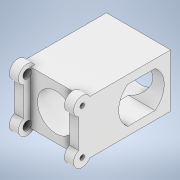
# Autodesk Inventor part: MotorMount
Saved by Autodesk Inventor 2022 (Build 260153000, 153)
## iProperties
Created: 2022-02-05
Part Number: MotorMount
Material: Generic
Document SubType Name: Modeling
Designer: ultra
Density: 1 g/cm^3
Appearance: Smooth - White
Author: ultra
Autodesk Inventor part; units mm, degrees
ref_plane "YZ Plane" through (0, 0, 0) normal (1, 0, 0) x (0, 1, 0)
ref_plane "XZ Plane" through (0, 0, 0) normal (0, 1, 0) x (-1, 0, 0)
ref_plane "XY Plane" through (0, 0, 0) normal (0, 0, 1) x (1, 0, 0)
sketch "Sketch1" plane through (0, 0, 0) normal (1, 0, 0) x (0, 1, 0)
  arc A0 (-5.7904, 15.7173) -> (3.1801, 16.4454) centre (0, 0) ccw
  line L0 (3.6239, 10.9763) -> (3.1801, 16.4454)
  line L1 (-5.3466, 10.2483) -> (3.6239, 10.9763)
  line L2 (-5.7904, 15.7173) -> (-5.3466, 10.2483)
  circle A1 centre (8.6526, -9.0212) radius 1.5
  circle A2 centre (-9.0212, -8.6526) radius 1.5
  circle A3 centre (-8.6526, 9.0212) radius 1.5
  circle A4 centre (9.0212, 8.6526) radius 1.5
  circle A5 centre (0, 0) radius 6.8
  circle A6 centre (8.6526, -9.0212) radius 1.5875
  circle A7 centre (-9.0212, -8.6526) radius 1.5875
  circle A8 centre (-8.6526, 9.0212) radius 1.5875
  circle A9 centre (9.0212, 8.6526) radius 1.5875
  circle A10 centre (0, 0) radius 16.75
  point P0 (-5.7904, 15.7173)
  point P1 (3.1801, 16.4454)
  dimension "d2" = 3.175
  dimension "d3" = 3.175
  dimension "d4" = 3.175
  dimension "d5" = 3.175
  constraints: 11 centre point, 6 end point, 5 coincident, 2 point on circle, 1 concentric
  measures "d2" diameter of A6
  measures "d3" diameter of A7
  measures "d4" diameter of A8
  measures "d5" diameter of A9
extrude "Extrusion3" add sketch "Sketch1" along normal blind 6.35 contours L2 L1 L0 A0 | A10 L0 L1 L2
sketch "Sketch4" plane through (6.35, 0, 0) normal (1, 0, 0) x (0, 0, -1)
  circle A0 centre (0, 0) radius 16.75 projected
  circle A1 centre (-25.4, 0) radius 6.35
  circle A2 centre (0, 0) radius 6.35
  circle A3 centre (-38.7858, -15.6249) radius 2.925
  circle A4 centre (-38.7858, 15.6249) radius 2.925
  line L0 (-41.275, 10.1656) -> (-41.275, -10.1656)
  arc A5 (-41.275, -10.1656) -> (-33.5216, -18.5039) centre (-38.7858, -15.6249) ccw
  line L1 (-33.5216, -18.5039) -> (20.3643, -18.5039)
  line L2 (-33.5216, 18.5039) -> (9.525, 18.5039)
  arc A6 (-33.5216, 18.5039) -> (-41.275, 10.1656) centre (-38.7858, 15.6249) ccw
  line L3 (20.3643, -18.5039) -> (20.3643, 18.5039)
  line L4 (20.3643, 18.5039) -> (8.806, 18.5039)
  point P0 (-41.275, 18.5039)
  constraints: 10 end point, 6 centre point, 4 point on circle, 1 point on line, 1 vertical
extrude "Extrusion5" add sketch "Sketch4" along normal blind 41.5544 contours A6 L2 L4 L3 L1 A5 L0
sketch "Sketch5" plane through (6.35, -18.5039, -20.3643) normal (0, 0, -1) x (-1, 0, 0)
  circle A0 centre (-20.7772, 18.5039) radius 12.8778
  point P0 (6.35, 18.5039)
  dimension "d22" = 25.7556
  constraints: 1 centre point
  measures "d22" diameter of A0
extrude "Extrusion6" cut sketch "Sketch5" against normal up to surface (61.6393 mm away)
sketch "Sketch6" plane through (6.35, 0, 0) normal (-1, 0, 0) x (0, 0, 1)
  circle A0 centre (25.4, 0) radius 6.35 projected
  circle A1 centre (38.7858, -15.6249) radius 2.925 projected
  circle A2 centre (38.7858, 15.6249) radius 2.925 projected
  line L0 (55.9002, 27.2812) -> (18.3497, 27.2812)
  line L1 (18.3497, 27.2812) -> (18.3497, -27.035)
  line L2 (18.3497, -27.035) -> (55.9002, -27.035)
  line L3 (55.9002, -27.035) -> (55.9002, 27.2812)
  constraints: 8 end point, 2 parallel, 1 horizontal, 1 perpendicular
extrude "Extrusion7" cut sketch "Sketch6" against normal blind 76.2
sketch "Sketch7" plane through (6.35, -18.5039, 18.3497) normal (0, 0, 1) x (1, 0, 0)
  line L0 (41.5544, 0) -> (0, 0) projected
  line L1 (41.5544, 37.0078) -> (41.5544, 0) projected
  line L2 (0, 37.0078) -> (41.5544, 37.0078) projected
  line L3 (0, 0) -> (0, 37.0078) projected
  circle A0 centre (20.7772, 18.5039) radius 12.8778 projected
  point P0 (-6.35, 18.5039)
extrude "Extrusion8" add sketch "Sketch7" along normal blind 25.4
sketch "Sketch8" plane through (6.35, 0, 0) normal (-1, 0, 0) x (0, 0, 1)
  line L0 (43.7497, -18.5039) -> (-17.8897, -18.5039)
  line L1 (43.7497, 18.5039) -> (43.7497, -18.5039)
  line L2 (-7.0503, 18.5039) -> (43.7497, 18.5039)
  line L3 (-25.5542, 0.0039) -> (43.7497, 0.0039)
  line L4 (43.7497, 12.8817) -> (43.7497, -12.8739)
  circle A0 centre (41.2605, -15.6249) radius 1.5875
  circle A1 centre (41.2605, 15.6249) radius 1.5875
  dimension "d29" = 3.175
  dimension "d30" = 3.175
  dimension "d31" = 2.7432
  dimension "d32" = 2.4892
  dimension "d33" = 2.879
  dimension "d34" = 2.879
  constraints: 10 end point, 2 centre point, 1 midpoint
  measures "d29" diameter of A0
  measures "d30" diameter of A1
  measures "d31" vertical distance of L4.start A1.centre
  measures "d32" distance from line of L1 A0.centre
  measures "d33" distance from line of L0 A0.centre
  measures "d34" distance from line of L2 A1.centre
extrude "Extrusion9" cut sketch "Sketch8" against normal blind 50.8
sketch "Sketch9" plane through (0, 0, 0) normal (-1, 0, 0) x (0, 0, 1)
  circle A0 centre (0, 0) radius 16.75 projected
  circle A1 centre (8.6526, 9.0212) radius 1.5875 projected
  circle A2 centre (9.0212, -8.6526) radius 1.5875 projected
  circle A3 centre (-8.6526, -9.0212) radius 1.5875 projected
  circle A4 centre (-9.0212, 8.6526) radius 1.5875 projected
  circle A5 centre (0, 0) radius 6.8 projected
sketch "Sketch10" plane through (6.35, 0, 0) normal (-1, 0, 0) x (0, 0, 1)
  circle A0 centre (41.2605, 15.6249) radius 1.5875 projected
  circle A1 centre (41.2605, -15.6249) radius 1.5875 projected
  circle A2 centre (0, 0) radius 16.75 projected
  line L0 (-20.3643, 18.5039) -> (43.7497, 18.5039) projected
  line L1 (-20.3643, -18.5039) -> (-20.3643, 18.5039) projected
  line L2 (43.7497, -18.5039) -> (-20.3643, -18.5039) projected
  line L3 (43.7497, 18.5039) -> (43.7497, -18.5039) projected
extrude "Extrusion10" add sketch "Sketch10" along normal blind 3.175
extrude "Extrusion11" cut sketch "Sketch9" against normal blind 3.175
sketch "Sketch11" plane through (6.35, 0, 0) normal (1, 0, 0) x (0, 0, -1)
  circle A0 centre (0, 0) radius 16.75 projected
  circle A1 centre (-8.6526, 9.0212) radius 1.5875 projected
  circle A2 centre (-9.0212, -8.6526) radius 1.5875 projected
  circle A3 centre (8.6526, -9.0212) radius 1.5875 projected
  circle A4 centre (9.0212, 8.6526) radius 1.5875 projected
  circle A5 centre (0, 0) radius 6.8 projected
extrude "Extrusion12" add sketch "Sketch11" along normal blind 3.175
sketch "Sketch12" plane through (3.175, 0, 0) normal (-1, 0, 0) x (0, 0, 1)
  circle A0 centre (41.2605, -15.6249) radius 1.5875 projected
  circle A1 centre (41.2605, 15.6249) radius 1.5875 projected
  circle A2 centre (41.2605, 15.6249) radius 6
  circle A3 centre (41.2605, -15.6249) radius 6
  dimension "d43" = 12
  dimension "d44" = 12
  constraints: 2 centre point, 2 coincident
  measures "d43" diameter of A2
  measures "d44" diameter of A3
sketch "Sketch13" plane through (47.9044, 0, 0) normal (1, 0, 0) x (0, 0, -1)
  circle A0 centre (-41.2605, 15.6249) radius 1.5875 projected
  circle A1 centre (-41.2605, -15.6249) radius 1.5875 projected
  circle A2 centre (-41.2605, -15.6249) radius 6
  circle A3 centre (-41.2605, 15.6249) radius 6
  constraints: 2 centre point, 2 coincident
sketch "Sketch14" plane through (6.35, -18.5039, 43.7497) normal (0, 0, 1) x (1, 0, 0)
  line L0 (36.7792, 28.6695) -> (36.7792, 37.0078) projected
  line L1 (41.5544, 37.0078) -> (-3.175, 37.0078) projected
  line L2 (1.6002, 37.0078) -> (1.6002, 28.6695) projected
  line L3 (1.6002, 28.6695) -> (-3.175, 28.6695) projected
  line L4 (-3.175, 0) -> (-3.175, 37.0078) projected
  line L5 (-3.175, 8.3383) -> (1.6002, 8.3383) projected
  line L6 (1.6002, 8.3383) -> (1.6002, 0) projected
  line L7 (41.5544, 0) -> (-3.175, 0) projected
  line L8 (36.7792, 0) -> (36.7792, 8.3383) projected
  line L9 (36.7792, 8.3383) -> (41.5544, 8.3383) projected
  line L10 (41.5544, 0) -> (41.5544, 37.0078) projected
  line L11 (41.5544, 28.6695) -> (36.7792, 28.6695) projected
  circle A0 centre (20.7772, 18.5039) radius 12.8778 projected
  point P0 (-6.35, 18.5039)
extrude "Extrusion15" cut sketch "Sketch14" against normal blind 5.0038 contours L11 L10 L9 L8 L7 L6 L5 L4 L3 L2 L1 L0
extrude "Extrusion16" add sketch "Sketch13" against normal blind 4.7752
extrude "Extrusion17" add sketch "Sketch12" against normal blind 4.7752
sketch "Sketch15" plane through (3.175, 0, 0) normal (-1, 0, 0) x (0, 0, 1)
  circle A0 centre (41.2605, -15.6249) radius 1.5875 projected
  circle A1 centre (41.2605, 15.6249) radius 1.5875 projected
  arc A2 (38.7713, 10.1656) -> (35.9963, 18.5039) centre (41.2605, 15.6249) ccw projected
  arc A3 (35.9963, -18.5039) -> (38.7713, -10.1656) centre (41.2605, -15.6249) ccw projected
  circle A4 centre (41.2605, -15.6249) radius 2.925
  circle A5 centre (41.2605, 15.6249) radius 2.925
  dimension "d55" = 5.85
  dimension "d56" = 5.85
  constraints: 2 centre point, 2 coincident
  measures "d55" diameter of A4
  measures "d56" diameter of A5
extrude "Extrusion18" cut sketch "Sketch15" against normal blind 6.6675
sketch "Sketch16" plane through (3.175, 0, 0) normal (-1, 0, 0) x (0, 0, 1)
  line L0 (38.7713, -10.1656) -> (38.7459, -10.1656) projected
  line L1 (38.7459, -10.1656) -> (38.7459, 10.1656) projected
  line L2 (38.7459, 10.1656) -> (38.7713, 10.1656) projected
  arc A0 (38.7713, 10.1656) -> (35.9963, 18.5039) centre (41.2605, 15.6249) ccw projected
  arc A1 (35.9963, -18.5039) -> (38.7713, -10.1656) centre (41.2605, -15.6249) ccw projected
  circle A2 centre (41.2605, 15.6249) radius 1.5875
  circle A3 centre (41.2605, -15.6249) radius 1.5875
  line L3 (-20.3643, 18.5039) -> (43.7497, 18.5039)
  line L4 (43.7497, -18.5039) -> (-20.3643, -18.5039)
  line L5 (43.7497, 18.5039) -> (43.7497, -18.5039)
  line L6 (38.7459, -18.5039) -> (35.9963, -18.5039) projected
  line L7 (38.3355, -18.5039) -> (38.3355, 18.5039)
  point P0 (43.7497, -10.1656)
  point P1 (43.7497, 10.1656)
  constraints: 8 end point, 2 centre point, 2 point on line, 1 perpendicular
extrude "Extrusion19" add sketch "Sketch16" against normal blind 4.7752 contours L0 L1 L2 A0 L5 A1
sketch "Sketch17" plane through (47.9044, 0, 0) normal (1, 0, 0) x (0, 0, -1)
  line L0 (-38.7713, 10.1656) -> (-38.7459, 10.1656) projected
  line L1 (-38.7459, 10.1656) -> (-38.7459, -10.1656) projected
  line L2 (-38.7459, -10.1656) -> (-38.7713, -10.1656) projected
  arc A0 (-38.7713, -10.1656) -> (-35.9963, -18.5039) centre (-41.2605, -15.6249) ccw projected
  arc A1 (-35.9963, 18.5039) -> (-38.7713, 10.1656) centre (-41.2605, 15.6249) ccw projected
  circle A2 centre (-41.2605, -15.6249) radius 1.5875
  circle A3 centre (-41.2605, 15.6249) radius 1.5875
  line L3 (20.3643, -18.5039) -> (-43.7497, -18.5039)
  line L4 (-43.7497, 18.5039) -> (20.3643, 18.5039)
  line L5 (-43.7497, -18.5039) -> (-43.7497, 18.5039)
  point P0 (-43.7497, 10.1656)
  point P1 (-43.7497, -10.1656)
  constraints: 6 end point, 2 centre point
extrude "Extrusion20" add sketch "Sketch17" against normal blind 4.7752 contours L0 L1 L2 A0 L5 A1
sketch "Sketch18" plane through (7.9502, 18.5039, 38.7459) normal (1, 0, 0) x (0, 0, -1)
  arc A0 (0, -32.6347) -> (0, -35.6229) centre (-2.5146, -34.1288) ccw projected
  arc A1 (0, -1.3849) -> (0, -4.3731) centre (-2.5146, -2.879) ccw projected
  line L0 (0, -1.3849) -> (0, 0) projected
  line L1 (2.7496, 0) -> (0, 0) projected
  arc A2 (2.7496, 0) -> (-5.0038, -8.3383) centre (-2.5146, -2.879) ccw projected
  line L2 (-5.0038, -8.3383) -> (-5.0038, -28.6695) projected
  arc A3 (-5.0038, -28.6695) -> (2.7496, -37.0078) centre (-2.5146, -34.1288) ccw projected
  line L3 (0, -37.0078) -> (2.7496, -37.0078) projected
  line L4 (0, -37.0078) -> (0, -4.3731) projected
  point P0 (38.7459, -18.5039)
  point P1 (0, -32.6347)
sketch "Sketch19" plane through (43.1292, -18.5039, 38.7459) normal (-1, 0, 0) x (0, 0, 1)
  circle A0 centre (2.5146, 2.879) radius 1.5875 projected
  circle A1 centre (2.5146, 34.1288) radius 1.5875 projected
  line L0 (0, 37.0078) -> (0, 0) projected
  line L1 (-2.7496, 0) -> (0, 0) projected
  arc A2 (-2.7496, 0) -> (5.0038, 8.3383) centre (2.5146, 2.879) ccw projected
  line L2 (5.0038, 8.3383) -> (5.0038, 28.6695) projected
  arc A3 (5.0038, 28.6695) -> (-2.7496, 37.0078) centre (2.5146, 34.1288) ccw projected
  line L3 (0, 37.0078) -> (-2.7496, 37.0078) projected
  point P0 (-38.7459, 18.5039)
extrude "Extrusion22" add sketch "Sketch19" along normal blind 1.5875
extrude "Extrusion23" add sketch "Sketch18" along normal blind 1.5875 contours A0 L4 L3 A3 L2 A2 L1 L0 A1
sketch "Sketch20" plane through (9.525, 0, 0) normal (1, 0, 0) x (0, 0, -1)
  circle A0 centre (0, 0) radius 16.75 projected
  circle A1 centre (0, 0) radius 6.8 projected
  circle A2 centre (8.6526, -9.0212) radius 1.5875 projected
  circle A3 centre (-9.0212, -8.6526) radius 1.5875 projected
  circle A4 centre (-8.6526, 9.0212) radius 1.5875 projected
  circle A5 centre (-8.6526, 9.0212) radius 3.175
  circle A6 centre (9.0212, 8.6526) radius 1.5875 projected
  circle A7 centre (9.0212, 8.6526) radius 3.175
  circle A8 centre (8.6526, -9.0212) radius 3.175
  circle A9 centre (-9.0212, -8.6526) radius 3.175
  circle A10 centre (0, 0) radius 15.85
  dimension "d69" = 6.35
  dimension "d70" = 6.35
  dimension "d71" = 6.35
  dimension "d72" = 6.35
  constraints: 5 centre point, 5 coincident
  measures "d69" diameter of A5
  measures "d70" diameter of A7
  measures "d71" diameter of A8
  measures "d72" diameter of A9
sketch "Sketch21" plane through (47.9044, -18.5039, -20.3643) normal (0, 0, -1) x (-1, 0, 0)
  circle A0 centre (20.7772, 18.5039) radius 12.8778 projected
  point P0 (47.9044, 18.5039)
extrude "Extrusion26" add sketch "Sketch20" along normal up to surface (38.3794 mm away) contours A0
sketch "Sketch22" plane through (47.9044, 0, 0) normal (1, 0, 0) x (0, 0, -1)
  circle A0 centre (0, 0) radius 15.85 projected
  circle A1 centre (0, 0) radius 15.85 projected
  line L0 (0, 15.85) -> (0, 12.675)
  line L1 (0, 12.675) -> (-9.5167, 12.675)
  line L2 (0, 12.675) -> (9.5167, 12.675)
  line L3 (0, -15.85) -> (0, -12.675)
  line L4 (0, -12.675) -> (9.5167, -12.675)
  line L5 (0, -12.675) -> (-9.5167, -12.675)
  dimension "d79" = 3.175
  dimension "d80" = 3.175
  constraints: 12 end point, 6 point on circle, 2 perpendicular, 2 vertical, 1 horizontal, 1 point on line
  measures "d79" distance of L0.start L0.end
  measures "d80" distance of L3.start L3.end
extrude "Extrusion27" add sketch "Sketch22" against normal up to surface (38.3794 mm away) contours L2 L0 A0 | A0 L3 L4 | L0 L1 A0 | A0 L5 L3
extrude "Extrusion28" cut sketch "Sketch21" against normal blind 76.2
sketch "Sketch23" plane through (9.525, 0, 0) normal (1, 0, 0) x (0, 0, -1)
  circle A0 centre (9.0212, 8.6526) radius 1.5875 projected
  circle A1 centre (8.6526, -9.0212) radius 1.5875 projected
  circle A2 centre (-9.0212, -8.6526) radius 1.5875 projected
  circle A3 centre (-8.6526, 9.0212) radius 1.5875 projected
  circle A4 centre (-8.6526, 9.0212) radius 1.7145
  circle A5 centre (9.0212, 8.6526) radius 1.7145
  circle A6 centre (8.6526, -9.0212) radius 1.7145
  circle A7 centre (-9.0212, -8.6526) radius 1.5875 projected
  circle A8 centre (-9.0212, -8.6526) radius 1.7145
  dimension "d85" = 3.429
  dimension "d86" = 3.429
  dimension "d87" = 3.429
  dimension "d88" = 3.429
  constraints: 4 centre point, 4 coincident
  measures "d85" diameter of A4
  measures "d86" diameter of A5
  measures "d87" diameter of A6
  measures "d88" diameter of A8
extrude "Extrusion29" cut sketch "Sketch23" against normal blind 25.4 contours A0 | A4 | A6 | A8
body "Solid3"
